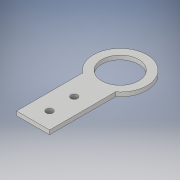
# Autodesk Inventor part: base gear connector
Saved by Autodesk Inventor 2018 (Build 220112000, 112)
## iProperties
Created: 2019-01-25
Part Number: base gear connector
Material: Generic
Document SubType Name: Modeling
Designer: s-2513225
Density: 1 g/cm^3
Appearance: Default
Author: s-2513225
Autodesk Inventor part; units mm, degrees
ref_plane "YZ Plane" through (0, 0, 0) normal (1, 0, 0) x (0, 1, 0)
ref_plane "XZ Plane" through (0, 0, 0) normal (0, 1, 0) x (-1, 0, 0)
ref_plane "XY Plane" through (0, 0, 0) normal (0, 0, 1) x (1, 0, 0)
sketch "Sketch1" plane through (0, 0, 0) normal (0, 1, 0) x (-1, 0, 0)
  line L0 (0, 0) -> (25.4, 0)
  line L1 (25.4, 0) -> (25.4, -50.8)
  line L2 (0, -50.8) -> (0, 0)
  circle A0 centre (12.7, -67.2144) radius 14.2875
  arc A1 (0.191, -50.8) -> (25.209, -50.8) centre (12.7, -67.2144) ccw
  line L3 (25.4, -50.8) -> (25.209, -50.8)
  line L4 (0.191, -50.8) -> (0, -50.8)
  line L5 (12.7, 0) -> (12.7, -12.7) construction
  line L6 (12.7, -12.7) -> (12.7, -31.75) construction
  circle A2 centre (12.7, -12.7) radius 2.5797
  circle A3 centre (12.7, -31.75) radius 2.5797
  dimension "d0" = 25.4
  dimension "d1" = 50.8
  dimension "d2" = 28.575
  dimension "d3" = 6.35
  dimension "d4" = 12.7
  dimension "d5" = 19.05
  dimension "d6" = 5.1594
  dimension "d7" = 5.1594
  constraints: 14 end point, 4 centre point, 3 parallel, 2 coincident, 2 point on circle, 1 horizontal, 1 midpoint, 1 perpendicular, 1 point on line, 1 vertical
  measures "d0" distance of L1.end L2.start
  measures "d1" distance of L0.end L1.end
  measures "d2" diameter of A0
  measures "d3" radial gap between concentric circles of A0 A1
  measures "d4" distance of L5.start L5.end
  measures "d5" distance of L5.end L6.end
  measures "d6" diameter of A2
  measures "d7" diameter of A3
extrude "Extrusion1" add sketch "Sketch1" along normal blind 3.175
body "Solid1"
